Autodesk Fusion 360 part; units mm, degrees
(part 2 of 2)
  spline S44 degree 2 poles (-28.6507, -24.1347) (-29.8115, -24.1371) (-30.4653, -23.6515) knots 0 0 0 1 1 1
  arc A18 (64.0367, -66.674) -> (63.5187, -65.7092) centre (63.7777, -66.1916) ccw
  line L162 (-31.3909, -21.1424) -> (-31.396, -18.6591)
  line L163 (-20.2167, -14.2211) -> (-20.2167, -14.0211)
  line L164 (-32.5375, -24.0363) -> (-33.7962, -24.0388)
  line L165 (-28.678, -21.1369) -> (-31.3909, -21.1424)
  spline S45 degree 5 poles (50.9366, -22.8645) (50.9348, -22.8259) (50.9292, -22.75) (50.9148, -22.6405) (50.8834, -22.5031) (50.8225, -22.3468) (50.738, -22.2071) (50.6282, -22.0855) (50.4922, -21.9825) (50.3313, -21.8972) (50.1475, -21.8281) (49.9836, -21.7847) (49.8519, -21.7585) (49.7602, -21.7438) (49.7134, -21.7371) knots 0 0 0 0 0 0 0.1 0.2 0.3 0.4 0.5 0.6 0.7 0.8 0.9 1 1 1 1 1 1
  line L166 (-18.5375, -12.7629) -> (-18.6809, -12.6194)
  line L167 (48.4274, -26.3644) -> (48.793, -25.0449)
  line L168 (50.9287, -28.6142) -> (49.4213, -28.6142)
  arc A19 (57.5739, -61.8275) -> (56.4337, -61.8275) centre (57.0038, -61.8275) ccw
  line L169 (-17.0167, -15.1211) -> (-17.0167, -14.2211)
  spline S46 degree 2 poles (-33.8519, -19.6208) (-33.9334, -19.2382) (-34.2379, -19.0071) knots 0 0 0 1 1 1
  line L170 (50.0446, -26.3644) -> (48.4274, -26.3644)
  line L171 (-18.9584, -12.7629) -> (-18.8149, -12.6194)
  line L172 (57.0038, -59.0823) -> (51.6038, -59.0823)
  line L173 (51.6038, -60.2085) -> (57.0038, -60.2085)
  spline S47 degree 2 poles (-25.5615, -20.9265) (-25.5595, -21.9003) (-25.9662, -22.658) knots 0 0 0 1 1 1
  line L174 (64.8038, -70.4149) -> (58.1231, -70.4149)
  line L175 (-20.4792, -14.2211) -> (-20.2167, -14.2211)
  line L176 (-17.2792, -14.2211) -> (-17.2792, -14.0211)
  spline S48 degree 2 poles (-29.4415, -18.9209) (-29.8388, -19.0769) (-30.1232, -19.2986) knots 0 0 0 1 1 1
  line L177 (63.7777, -66.1916) -> (60.0038, -68.2176) construction
  line L178 (49.078, -17.2) -> (47.7162, -22.4312)
  spline S49 degree 2 poles (-31.396, -18.6591) (-31.0013, -18.2755) (-30.2513, -17.9827) knots 0 0 0 1 1 1
  spline S50 degree 5 poles (50.9366, -22.8645) (50.9348, -22.8259) (50.9292, -22.75) (50.9148, -22.6405) (50.8834, -22.5031) (50.8225, -22.3468) (50.738, -22.2071) (50.6282, -22.0855) (50.4922, -21.9825) (50.3313, -21.8972) (50.1475, -21.8281) (49.9836, -21.7847) (49.8519, -21.7585) (49.7602, -21.7438) (49.7134, -21.7371) knots 0 0 0 0 0 0 0.1 0.2 0.3 0.4 0.5 0.6 0.7 0.8 0.9 1 1 1 1 1 1
  line L179 (49.4213, -28.6142) -> (50.0446, -26.3644)
  arc A20 (56.4337, -68.8176) -> (57.5739, -68.8176) centre (57.0038, -68.8176) ccw
  line L180 (57.0038, -68.8176) -> (57.0038, -61.8275) construction
  spline S51 degree 2 poles (-28.6528, -23.0589) (-27.8279, -23.0572) (-27.3421, -22.5332) knots 0 0 0 1 1 1
  line L181 (56.4337, -61.8275) -> (56.4337, -68.8176)
  line L182 (-31.3078, -22.3074) -> (-30.0581, -22.071)
  arc A21 (57.0038, -60.2085) -> (57.0038, -59.0823) centre (57.0038, -59.6454) ccw
  line L183 (-17.0167, -15.5211) -> (-17.2792, -15.5211)
  spline S52 degree 2 poles (-25.9662, -22.658) (-26.3729, -23.4158) (-27.1587, -23.8213) knots 0 0 0 1 1 1
  line L184 (50.4816, -66.7499) -> (53.8101, -68.7056)
  arc A22 (58.1231, -70.4149) -> (58.1231, -71.5881) centre (58.1231, -71.0015) ccw
  arc A23 (53.8101, -68.7056) -> (54.5831, -67.39) centre (54.1966, -68.0478) ccw
  spline S53 degree 2 poles (-28.7317, -17.6884) (-27.7537, -17.6864) (-27.0257, -18.0953) knots 0 0 0 1 1 1
  line L185 (52.5226, -22.8607) -> (50.9287, -28.6142)
  spline S54 degree 2 poles (-63.4491, -19.0533) (-63.7208, -19.2728) (-63.7754, -19.5919) knots 0 0 0 1 1 1
  line L186 (-70.944, -17.8799) -> (-65.8795, -17.8697)
  line L187 (-63.8286, -20.6508) -> (-63.8216, -24.0994)
  spline S55 degree 2 poles (-63.7754, -19.5919) (-63.8301, -19.9109) (-63.8286, -20.6508) knots 0 0 0 1 1 1
  line L188 (-65.8795, -17.8697) -> (-65.8773, -19.005)
  line L189 (-69.1434, -23.0556) -> (-66.239, -23.0497)
  line L190 (-66.2369, -24.1043) -> (-70.7996, -24.1135)
  line L191 (-63.8216, -24.0994) -> (-65.0803, -24.1019)
  spline S56 degree 2 poles (-64.6133, -18.4582) (-64.3397, -18.1387) (-63.8808, -17.9485) knots 0 0 0 1 1 1
  line L192 (-66.239, -23.0497) -> (-66.2369, -24.1043)
  line L193 (-65.0803, -24.1019) -> (-65.0869, -20.8277)
  spline S57 degree 2 poles (-65.0869, -20.8277) (-65.0892, -19.7051) (-64.988, -19.2414) knots 0 0 0 1 1 1
  line L194 (-67.3955, -18.923) -> (-70.9419, -18.9302)
  spline S58 degree 2 poles (-64.988, -19.2414) (-64.8869, -18.7776) (-64.6133, -18.4582) knots 0 0 0 1 1 1
  spline S59 degree 2 poles (-62.6416, -18.8327) (-63.1774, -18.8337) (-63.4491, -19.0533) knots 0 0 0 1 1 1
  spline S60 degree 5 poles (-17.0167, -17.9211) (-17.0192, -18.1019) (-17.0247, -18.4483) (-17.0348, -18.9224) (-17.0437, -19.4673) (-17.0058, -20.0268) (-16.8739, -20.4996) (-16.6158, -20.9275) (-16.2341, -21.3563) (-15.7621, -21.8302) (-15.2514, -22.3856) (-14.762, -23.0456) (-14.3504, -23.8136) (-14.0614, -24.6692) (-13.9287, -25.5763) (-13.9743, -26.4898) (-14.2086, -27.362) (-14.6299, -28.1493) (-15.2239, -28.82) (-15.9657, -29.3545) (-16.8219, -29.7417) (-17.7541, -29.9769) (-18.7208, -30.0593) (-19.6804, -29.9888) (-20.5934, -29.7639) (-21.4242, -29.384) (-22.141, -28.8524) (-22.7178, -28.1792) (-23.1347, -27.3841) (-23.3794, -26.5001) (-23.4479, -25.5734) (-23.346, -24.6548) (-23.0896, -23.7924) (-22.7069, -23.0242) (-22.2384, -22.3705) (-21.7396, -21.8252) (-21.2725, -21.3599) (-20.8919, -20.9331) (-20.6344, -20.4981) (-20.5035, -20.0118) (-20.4659, -19.4405) (-20.4724, -18.8956) (-20.4779, -18.4308) (-20.4792, -18.0953) (-20.4792, -17.9211) knots 0 0 0 0 0 0 0.025 0.05 0.075 0.1 0.125 0.15 0.175 0.2 0.225 0.25 0.275 0.3 0.325 0.35 0.375 0.4 0.425 0.45 0.475 0.5 0.525 0.55 0.575 0.6 0.625 0.65 0.675 0.7 0.725 0.75 0.775 0.8 0.825 0.85 0.875 0.9 0.925 0.95 0.975 1 1 1 1 1 1
  line L195 (-16.9853, -15.6382) -> (-17.0481, -20.2041)
  line L196 (-20.4792, -20.1211) -> (-20.4792, -15.7211)
  line L197 (-70.9419, -18.9302) -> (-70.944, -17.8799)
  line L198 (-70.7996, -24.1135) -> (-70.8016, -23.1354)
  line L199 (-51.6345, -24.0748) -> (-54.1432, -17.846)
  spline S61 degree 2 poles (-20.4647, -23.8375) (-20.2015, -23.5818) (-19.7016, -23.3866) knots 0 0 0 1 1 1
  line L200 (-50.9571, -22.6191) -> (-50.1198, -20.3042)
  spline S62 degree 2 poles (-19.5728, -26.1121) (-19.4843, -26.4181) (-19.2415, -26.5948) knots 0 0 0 1 1 1
  circle A24 centre (52.4889, -17.3797) radius 3.1155
  spline S63 degree 2 poles (-17.6398, -27.279) (-18.0391, -27.4868) (-18.6345, -27.488) knots 0 0 0 1 1 1
  spline S64 degree 2 poles (-17.7706, -24.2757) (-18.1002, -23.9064) (-18.6332, -23.9075) knots 0 0 0 1 1 1
  line L201 (-49.735, -19.2531) -> (-49.2233, -17.8361)
  spline S65 degree 2 poles (-17.5512, -23.4617) (-17.0659, -23.7343) (-16.821, -24.2426) knots 0 0 0 1 1 1
  spline S66 degree 2 poles (-16.575, -25.3491) (-16.5737, -25.9983) (-16.8448, -26.5035) knots 0 0 0 1 1 1
  line L202 (-47.8881, -17.8334) -> (-50.3036, -24.0721)
  spline S67 degree 2 poles (-19.7016, -23.3866) (-19.2016, -23.1914) (-18.6885, -23.1904) knots 0 0 0 1 1 1
  line L203 (-60.1094, -24.0919) -> (-61.368, -24.0944)
  line L204 (-54.1432, -17.846) -> (-52.774, -17.8432)
  line L205 (48.765, -61.1704) -> (45.6038, -61.1704) construction
  arc A25 (41.2766, -59.5046) -> (39.9627, -59.5046) centre (40.6197, -59.5046) ccw
  spline S68 degree 2 poles (-17.7621, -26.4203) (-17.4382, -26.0709) (-17.4396, -25.3849) knots 0 0 0 1 1 1
  circle A26 centre (56.0213, -23.5604) radius 3.0414
  line L206 (-60.1161, -20.7666) -> (-60.1094, -24.0919)
  arc A27 (38.4183, -62.0841) -> (36.1328, -68.1777) centre (38.3745, -65.5431) ccw
  line L207 (-65.8773, -19.005) -> (-69.1434, -23.0556)
  line L208 (-59.2311, -18.9066) -> (-59.2332, -17.8562)
  line L209 (-19.6151, -24.7911) -> (-18.6541, -24.7892)
  spline S69 degree 2 poles (-61.3749, -20.7181) (-61.3765, -19.9144) (-61.4237, -19.6764) knots 0 0 0 1 1 1
  line L210 (-50.3036, -24.0721) -> (-51.6345, -24.0748)
  line L211 (40.6197, -66.5435) -> (40.6197, -59.5046) construction
  spline S70 degree 2 poles (-18.6359, -26.7707) (-18.086, -26.7696) (-17.7621, -26.4203) knots 0 0 0 1 1 1
  arc A28 (36.1328, -68.1777) -> (37.0548, -67.0941) centre (36.5938, -67.6359) ccw
  line L212 (-20.4059, -26.2697) -> (-19.5728, -26.1121)
  line L213 (-56.091, -24.0328) -> (-56.1014, -18.9002)
  line L214 (-18.6527, -25.4894) -> (-20.4613, -25.4931)
  line L215 (42.4188, -59.63) -> (44.7886, -66.8332)
  line L216 (-54.8448, -17.8474) -> (-54.8324, -24.0302)
  spline S71 degree 2 poles (-16.821, -24.2426) (-16.5762, -24.751) (-16.575, -25.3491) knots 0 0 0 1 1 1
  line L217 (-49.2233, -17.8361) -> (-47.8881, -17.8334)
  line L218 (-61.368, -24.0944) -> (-61.3749, -20.7181)
  spline S72 degree 5 poles (44.3007, -16.8973) (44.3173, -16.863) (44.3472, -16.7953) (44.3822, -16.6962) (44.409, -16.5691) (44.4071, -16.4191) (44.3671, -16.2787) (44.2861, -16.1486) (44.1636, -16.0291) (44.002, -15.9194) (43.8046, -15.8188) (43.6205, -15.7449) (43.4687, -15.6929) (43.3615, -15.6597) (43.3064, -15.6436) knots 0 0 0 0 0 0 0.1 0.2 0.3 0.4 0.5 0.6 0.7 0.8 0.9 1 1 1 1 1 1
  line L219 (-59.2332, -17.8562) -> (-54.8448, -17.8474)
  line L220 (49.2038, -59.8176) -> (46.3446, -68.6318) construction
  line L221 (-18.6541, -24.7892) -> (-18.6527, -25.4894)
  arc A29 (36.8916, -59.1577) -> (36.0527, -59.6242) centre (36.4722, -59.3909) ccw
  line L222 (46.9604, -68.8315) -> (49.8196, -60.0174)
  circle A30 centre (41.0594, -15.5804) radius 1.0733
  spline S73 degree 2 poles (-19.1617, -24.012) (-19.4265, -24.1161) (-19.6162, -24.2639) knots 0 0 0 1 1 1
  line L223 (35.7794, -15.7004) -> (36.0194, -14.3804)
  line L224 (-19.6162, -24.2639) -> (-19.6151, -24.7911)
  arc A31 (45.7289, -68.432) -> (46.9604, -68.8315) centre (46.3446, -68.6318) ccw
  line L225 (-52.2268, -19.2581) -> (-49.735, -19.2531)
  arc A32 (40.6197, -69.3744) -> (40.6197, -68.2176) centre (40.6197, -68.796) ccw
  spline S74 degree 2 poles (-18.6885, -23.1904) (-18.0365, -23.1891) (-17.5512, -23.4617) knots 0 0 0 1 1 1
  spline S75 degree 2 poles (-18.6345, -27.488) (-19.4084, -27.4895) (-19.8442, -27.1658) knots 0 0 0 1 1 1
  spline S76 degree 2 poles (-61.4237, -19.6764) (-61.5053, -19.2939) (-61.8098, -19.0627) knots 0 0 0 1 1 1
  line L226 (44.5601, -22.3879) -> (42.7329, -22.3879)
  spline S77 degree 2 poles (-19.8442, -27.1658) (-20.28, -26.8421) (-20.4059, -26.2697) knots 0 0 0 1 1 1
  spline S78 degree 2 poles (-35.1102, -17.7013) (-34.2172, -17.6995) (-33.7554, -17.9048) knots 0 0 0 1 1 1
  line L227 (-52.774, -17.8432) -> (-52.2268, -19.2581)
  circle A33 centre (39.0194, -15.5804) radius 0.4327
  line L228 (-54.8324, -24.0302) -> (-56.091, -24.0328)
  line L229 (42.8594, -24.2204) -> (41.6483, -24.5507)
  spline S79 degree 2 poles (-61.8098, -19.0627) (-62.1143, -18.8316) (-62.6416, -18.8327) knots 0 0 0 1 1 1
  line L230 (38.365, -62.7953) -> (36.4722, -59.3909) construction
  spline S80 degree 2 poles (-62.682, -17.7569) (-61.7891, -17.7551) (-61.3273, -17.9604) knots 0 0 0 1 1 1
  arc A34 (44.7886, -66.8332) -> (45.836, -66.4886) centre (45.3123, -66.6609) ccw
  line L231 (-20.4613, -25.4931) -> (-20.4647, -23.8375)
  circle A35 centre (41.0594, -15.5804) radius 0.5367
  arc A36 (38.4003, -63.5068) -> (38.4183, -62.0841) centre (38.4093, -62.7955) ccw
  spline S81 degree 5 poles (35.364, -16.3525) (35.345, -16.369) (35.3063, -16.4012) (35.246, -16.4473) (35.1607, -16.5042) (35.0462, -16.5676) (34.924, -16.6224) (34.7945, -16.6675) (34.6587, -16.7009) (34.5181, -16.7199) (34.3747, -16.7214) (34.231, -16.703) (34.0895, -16.6628) (33.9528, -16.6008) (33.8236, -16.5191) (33.7043, -16.4212) (33.5971, -16.3111) (33.5039, -16.1933) (33.4262, -16.0715) (33.3645, -15.9482) (33.3191, -15.8248) (33.2959, -15.7266) (33.2857, -15.6534) (33.2822, -15.6047) (33.2812, -15.5804) knots 0 0 0 0 0 0 0.05 0.1 0.15 0.2 0.25 0.3 0.35 0.4 0.45 0.5 0.55 0.6 0.65 0.7 0.75 0.8 0.85 0.9 0.95 1 1 1 1 1 1
  spline S82 degree 2 poles (-17.4396, -25.3849) (-17.4411, -24.645) (-17.7706, -24.2757) knots 0 0 0 1 1 1
  arc A37 (38.4003, -63.5068) -> (37.0548, -67.0941) centre (38.3745, -65.5431) ccw
  spline S83 degree 2 poles (-35.8772, -18.9976) (-36.1489, -19.2172) (-36.2036, -19.5362) knots 0 0 0 1 1 1
  spline S84 degree 2 poles (-60.5969, -18.4947) (-60.3284, -18.8237) (-60.2426, -19.185) knots 0 0 0 1 1 1
  line L232 (37.3394, -16.0604) -> (37.8194, -14.5004)
  line L233 (-24.9205, -63.1597) -> (-27.0005, -64.4597) construction
  arc A38 (-24.4038, -63.9865) -> (-25.4373, -62.3329) centre (-24.9205, -63.1597) ccw
  line L234 (-24.1393, -69.2134) -> (-27.7794, -67.1334) construction
  line L235 (-23.6556, -68.3669) -> (-27.2956, -66.2868)
  line L236 (-37.0255, -65.8956) -> (-38.3784, -61.6815)
  arc A39 (-49.9858, -65.6876) -> (-48.5071, -66.1846) centre (-49.2464, -65.9361) ccw
  line L237 (-28.2631, -67.9799) -> (-24.623, -70.0599)
  arc A40 (-24.623, -70.0599) -> (-23.6556, -68.3669) centre (-24.1393, -69.2134) ccw
  line L238 (-41.1451, -59.5878) -> (-45.3305, -59.5878)
  line L239 (-26.4838, -65.2865) -> (-24.4038, -63.9865)
  line L240 (-44.0827, -70.774) -> (-47.9547, -68.0452)
  arc A41 (-46.9952, -61.6857) -> (-48.4739, -61.1888) centre (-47.7345, -61.4372) ccw
  arc A42 (-28.7358, -60.3803) -> (-30.6858, -60.3803) centre (-29.7108, -60.3803) ccw
  line L241 (-29.7108, -64.0124) -> (-29.7108, -60.3803) construction
  arc A43 (-28.6905, -69.3997) -> (-30.5105, -69.3997) centre (-29.6005, -69.3997) ccw
  line L242 (-30.5105, -69.3997) -> (-30.5105, -71.4797)
  line L243 (-42.0828, -71.2842) -> (-38.3358, -68.5989) construction
  line L244 (-28.6905, -71.4797) -> (-28.6905, -69.3997)
  arc A44 (-33.5901, -62.5982) -> (-34.6718, -64.2207) centre (-34.131, -63.4095) ccw
  line L245 (-49.2464, -65.9361) -> (-47.7345, -61.4372) construction
  line L246 (-48.4739, -61.1888) -> (-49.9858, -65.6876)
  line L247 (-25.4373, -62.3329) -> (-27.5173, -63.6329)
  line L248 (-34.6718, -64.2207) -> (-33.1118, -65.2608)
  arc A45 (-41.1451, -61.1478) -> (-41.1451, -59.5878) centre (-41.1451, -60.3678) ccw
  arc A46 (-37.8815, -69.2329) -> (-38.7902, -67.9649) centre (-38.3358, -68.5989) ccw
  line L249 (-32.0301, -63.6383) -> (-33.5901, -62.5982)
  arc A47 (-33.1118, -65.2608) -> (-32.0301, -63.6383) centre (-32.5709, -64.4495) ccw
  arc A48 (-44.9814, -72.0491) -> (-44.0827, -70.774) centre (-44.532, -71.4115) ccw
  line L250 (-34.5019, -70.2048) -> (-30.8619, -67.8647)
  arc A49 (-47.9547, -68.0452) -> (-48.8533, -69.3203) centre (-48.404, -68.6827) ccw
  line L251 (-31.9164, -66.2244) -> (-35.5564, -68.5645)
  line L252 (-48.5071, -66.1846) -> (-46.9952, -61.6857)
  line L253 (-37.7682, -66.134) -> (-39.1211, -61.92) construction
  arc A50 (-35.5564, -68.5645) -> (-34.5019, -70.2048) centre (-35.0291, -69.3846) ccw
  line L254 (-31.3891, -67.0445) -> (-35.0291, -69.3846) construction
  arc A51 (-30.6858, -64.0124) -> (-28.7358, -64.0124) centre (-29.7108, -64.0124) ccw
  arc A52 (-30.8619, -67.8647) -> (-31.9164, -66.2244) centre (-31.3891, -67.0445) ccw
  line L255 (-38.7902, -67.9649) -> (-42.5371, -70.6502)
  line L256 (-29.6005, -71.4797) -> (-29.6005, -69.3997) construction
  line L257 (-48.8533, -69.3203) -> (-44.9814, -72.0491)
  line L258 (-30.6858, -60.3803) -> (-30.6858, -64.0124)
  line L259 (-28.7358, -64.0124) -> (-28.7358, -60.3803)
  line L260 (-45.3305, -61.1478) -> (-41.1451, -61.1478)
  line L261 (-32.5709, -64.4495) -> (-34.131, -63.4095) construction
  arc A53 (-45.3305, -59.5878) -> (-45.3305, -61.1478) centre (-45.3305, -60.3678) ccw
  arc A54 (-38.3784, -61.6815) -> (-39.8637, -62.1584) centre (-39.1211, -61.92) ccw
  arc A55 (-30.5105, -71.4797) -> (-28.6905, -71.4797) centre (-29.6005, -71.4797) ccw
  line L262 (-41.6284, -71.9182) -> (-37.8815, -69.2329)
  arc A56 (-38.5109, -66.3725) -> (-37.0255, -65.8956) centre (-37.7682, -66.134) ccw
  arc A57 (-27.5173, -63.6329) -> (-26.4838, -65.2865) centre (-27.0005, -64.4597) ccw
  line L263 (-39.8637, -62.1584) -> (-38.5109, -66.3725)
  line L264 (-44.532, -71.4115) -> (-48.404, -68.6827) construction
  arc A58 (-42.5371, -70.6502) -> (-41.6284, -71.9182) centre (-42.0828, -71.2842) ccw
  line L265 (-41.1451, -60.3678) -> (-45.3305, -60.3678) construction
  arc A59 (-27.2956, -66.2868) -> (-28.2631, -67.9799) centre (-27.7794, -67.1334) ccw
  line L266 (88.5, -105.5) -> (85.5, -105.5)
  line L267 (85.5, -105.5) -> (85.5, -9.5)
  line L268 (85.5, -9.5) -> (88.5, -9.5)
  line L269 (88.5, -9.5) -> (88.5, -105.5)
  line L270 (-88.5, -9.5) -> (-88.5, -105.5)
  line L271 (-85.5, -105.5) -> (-85.5, -9.5)
  line L272 (28, -111) -> (-28, -111)
  line L273 (-51, -103) -> (-61, -103)
  line L274 (-61, -103) -> (-61, -111)
  line L275 (-61, -111) -> (-51, -111)
  line L276 (-51, -111) -> (-51, -103)
  line L277 (-28, -111) -> (-56, -111)
  line L278 (90, -4) -> (84, -4)
  line L279 (84, -4) -> (84, -4.5)
  line L280 (84, -4.5) -> (90, -4.5)
  line L281 (90, -4.5) -> (90, -4)
  line L282 (90, -111) -> (84, -111)
  line L283 (84, -111) -> (84, -110.5)
  line L284 (84, -110.5) -> (90, -110.5)
  line L285 (90, -110.5) -> (90, -111)
  line L286 (-84, -110.5) -> (-90, -110.5)
  line L287 (-84, -4.5) -> (-90, -4.5)
  line L288 (84, -4.5) -> (-84, -4.5)
  line L289 (-84, -110.5) -> (84, -110.5)
  point P0 (61.02, -25.7233)
  point P1 (46.5762, -56.9164)
  point P2 (46.0215, -56.8133)
  point P3 (46.9394, -27.3404)
  point P4 (33.4994, -16.1804)
  point P5 (-14.3792, -27.6211)
  point P6 (-14.8792, -22.9211)
  point P7 (44.0594, -27.2628)
  point P8 (60.3867, -21.4673)
  point P9 (45.7317, -28.1654)
  point P10 (36.0194, -16.0142)
  point P11 (35.8994, -16.6605)
  point P12 (34.0914, -15.7841)
  point P13 (51.444, -20.7686)
  point P14 (63.9087, -20.9288)
  point P15 (44.7794, -28.5404)
  point P16 (37.3394, -16.6604)
  point P17 (43.4594, -28.3004)
  point P18 (34.8065, -16.6605)
  point P19 (57.9901, -18.9866)
  point P20 (-20.7292, -20.6211)
  point P21 (-22.5675, -22.8627)
  point P22 (-18.7792, -30.0211)
  point P23 (-22.9792, -27.6211)
  point P24 (-16.7792, -20.6211)
  point P25 (34.3141, -16.0142)
  point P26 (36.4355, -16.0142)
  point P27 (52.3172, -21.7688)
  point P28 (34.8282, -15.7841)
  point P29 (37.413, -16.3545)
  point P30 (50.6346, -22.1023)
  point P31 (44.9249, -27.2628)
  point P32 (34.0994, -16.6605)
  point P33 (44.3007, -16.184)
  point P34 (45.922, -16.1545)
  point P35 (48.6673, -15.0707)
  point P36 (47.4568, -16.2272)
  point P37 (58.4309, -20.5116)
  point P38 (50.6346, -22.1023)
  point P39 (60.5566, -20.5116)
  point P40 (56.7906, -20.1404)
  point P41 (49.078, -16.1977)
  point P42 (49.8965, -23.22)
  point P43 (45.5113, -15.0275)
  point P44 (46.5762, -56.9164)
  point P45 (49.267, -68.4427)
  point P46 (46.5762, -56.9164)
  point P47 (62.2394, -20.5807)
  point P48 (36.4573, -16.6605)
  point P49 (59.5394, -24.3404)
  point P50 (-33.2091, -68.2146)
  point P51 (-48.4905, -63.6867)
  point P52 (-29.7108, -62.1964)
  point P53 (-46.468, -70.0471)
  point P54 (-38.4446, -64.027)
  point P55 (-33.3509, -63.9295)
  point P56 (-40.2093, -69.9415)
  point P57 (-25.9605, -63.8097)
  point P58 (-29.6005, -70.4397)
  point P59 (-36.6222, -66.278)
  point P60 (-25.9593, -68.1734)
  point P61 (-43.2378, -60.3678)
  dimension "d154" = 180
  dimension "d155" = 115
  dimension "d156" = 180
  dimension "d157" = 4
  dimension "d158" = 1.5
  dimension "d159" = 5.5
  dimension "d160" = 3
  dimension "d161" = 1.5
  dimension "d162" = 1.5
  dimension "d163" = 5.5
  dimension "d164" = 3
  dimension "d165" = 56
  dimension "d166" = 10
  dimension "d167" = 8
  dimension "d168" = 0.5
  dimension "d169" = 0.5
  constraint horizontal L4
  constraint vertical L5
  constraint horizontal L6
  constraint vertical L7
  constraint coincident L0.end L1.start
  constraint horizontal L8
  constraint vertical L9
  constraint horizontal L10
  constraint vertical L11
  constraint perpendicular L5 L12
  constraint perpendicular L10 L13
  constraint perpendicular L13 L14
  constraint coincident L10 L15.end
  constraint perpendicular L10 L15
  constraint coincident L10 L16.end
  constraint coincident L2 L17.end
  constraint perpendicular L2 L17
  constraint coincident L2.end L3.start
  constraint coincident L2 L18.end
  constraint perpendicular L18 L19
  constraint perpendicular L19 L20
  constraint coincident L2 L21.end
  constraint perpendicular L2 L21
  constraint symmetric L12.end L23 L28.start
  constraint symmetric L13.end L23 L27.start
  constraint symmetric L14.end L23 L26.start
  constraint symmetric L15.end L23 L25.start
  constraint symmetric L16.end L23 L24.start
  constraint symmetric L17.end L23 L24.end
  constraint symmetric L2.end L23 L1.end
  constraint symmetric L18.end L23 L29.end
  constraint symmetric L19.end L23 L30.end
  constraint symmetric L20.end L23 L31.end
  constraint symmetric L21.end L23 L32.end
  constraint parallel L179 L185
  constraint parallel L168 L170
  constraint parallel L167 L185
  constraint parallel L156 L170
  constraint parallel L142 L167
  constraint perpendicular L117 L123
  constraint perpendicular L93 L117
  constraint perpendicular L88 L229
  constraint perpendicular L56 L229
  constraint concentric A30 A35
  constraint coincident L79.start A35
  constraint coincident L79.end A30
  constraint coincident L106.start A35
  constraint coincident L106.end A30
  constraint perpendicular L79 L106
  constraint concentric A0 A33
  constraint parallel L71 L232
  constraint parallel L101 L223
  constraint parallel L57 L59
  constraint parallel L58 L101
  constraint midpoint P49 L68
  constraint tangent L145 A17
  constraint tangent L127 A17
  constraint parallel L127 L145
  constraint tangent L127 A15
  constraint tangent A15 L145
  constraint tangent A4 L83
  constraint tangent A4 L76
  constraint parallel L76 L83
  constraint tangent L76 A11
  constraint tangent L83 A11
  constraint tangent L121 A16
  constraint tangent A16 L184
  constraint parallel L121 L184
  constraint tangent L184 A23
  constraint tangent L121 A23
  constraint tangent L134 A19
  constraint tangent A19 L181
  constraint parallel L134 L181
  constraint tangent A20 L181
  constraint tangent L134 A20
  constraint tangent A14 L150
  constraint tangent A14 L147
  constraint parallel L147 L150
  constraint tangent L147 A18
  constraint tangent L150 A18
  constraint tangent L89 A12
  constraint tangent A12 L174
  constraint parallel L89 L174
  constraint tangent L174 A22
  constraint tangent L89 A22
  constraint perpendicular L126 L134
  constraint tangent A13 L172
  constraint tangent A13 L173
  constraint parallel L172 L173
  constraint tangent L173 A21
  constraint tangent L172 A21
  constraint perpendicular L130 L134
  constraint tangent L116 A31
  constraint tangent L222 A31
  constraint parallel L116 L222
  constraint tangent A9 L222
  constraint tangent A9 L116
  constraint tangent L80 A10
  constraint tangent L55 A10
  constraint parallel L55 L80
  constraint tangent L55 A5
  constraint tangent A5 L80
  constraint coincident A5.centre L220
  constraint tangent A1 L105
  constraint tangent A1 L215
  constraint parallel L105 L215
  constraint tangent L215 A34
  constraint tangent L105 A34
  constraint tangent L110 A25
  constraint tangent L61 A25
  constraint parallel L61 L110
  constraint tangent L61 A6
  constraint tangent A6 L110
  constraint tangent A3 L48
  constraint tangent L35 A3
  constraint parallel L35 L48
  constraint tangent L35 A32
  constraint tangent L48 A32
  constraint tangent A27 A36
  constraint tangent A36 A37
  constraint tangent A28 A37
  constraint tangent A27 A28
  constraint tangent L78 A29
  constraint tangent L64 A29
  constraint parallel L64 L78
  constraint tangent A2 L64
  constraint tangent A2 L78
  constraint coincident A2.centre A7
  constraint midpoint L109.end L196
  constraint midpoint L109.start L195
  constraint perpendicular L109 L196
  constraint coincident L45.end L196
  constraint perpendicular L45 L196
  constraint coincident L91.end L196
  constraint perpendicular L45 L113
  constraint perpendicular L115 L196
  constraint perpendicular L84 L115
  constraint perpendicular L84 L100
  constraint perpendicular L95 L100
  constraint perpendicular L95 L183
  constraint perpendicular L100 L124
  constraint perpendicular L124 L131
  constraint perpendicular L131 L169
  constraint perpendicular L124 L161
  constraint perpendicular L161 L176
  constraint parallel L146 L152
  constraint parallel L155 L159
  constraint parallel L125 L144
  constraint parallel L141 L157
  constraint parallel L159 L171
  constraint perpendicular L166 L171
  constraint parallel L151 L152
  constraint parallel L86 L148
  constraint parallel L43 L77
  constraint tangent A42 L259
  constraint tangent A42 L258
  constraint parallel L258 L259
  constraint tangent A51 L258
  constraint tangent A51 L259
  constraint midpoint P52 L241
  constraint tangent A44 L249
  constraint tangent A44 L248
  constraint parallel L248 L249
  constraint tangent L248 A47
  constraint tangent L249 A47
  constraint midpoint P55 L261
  constraint tangent L251 A50
  constraint tangent L250 A50
  constraint parallel L250 L251
  constraint tangent L250 A52
  constraint tangent L251 A52
  constraint midpoint P50 L254
  constraint tangent A43 L244
  constraint tangent A43 L242
  constraint parallel L242 L244
  constraint tangent L242 A55
  constraint tangent L244 A55
  constraint midpoint P58 L256
  constraint tangent L235 A59
  constraint tangent L237 A59
  constraint parallel L235 L237
  constraint tangent L237 A40
  constraint tangent L235 A40
  constraint midpoint P60 L234
  constraint tangent L247 A57
  constraint tangent L239 A57
  constraint parallel L239 L247
  constraint tangent A38 L239
  constraint tangent A38 L247
  constraint midpoint P57 L233
  constraint tangent A46 L262
  constraint tangent A46 L255
  constraint parallel L255 L262
  constraint tangent L255 A58
  constraint tangent L262 A58
  constraint midpoint P56 L243
  constraint tangent L236 A54
  constraint tangent A54 L263
  constraint parallel L236 L263
  constraint tangent A56 L263
  constraint tangent L236 A56
  constraint midpoint P54 L253
  constraint tangent L238 A53
  constraint tangent L260 A53
  constraint parallel L238 L260
  constraint tangent A45 L260
  constraint tangent L238 A45
  constraint midpoint P61 L265
  constraint tangent A41 L252
  constraint tangent A41 L246
  constraint parallel L246 L252
  constraint tangent A39 L246
  constraint tangent A39 L252
  constraint midpoint P51 L245
  constraint tangent L240 A49
  constraint tangent A49 L257
  constraint parallel L240 L257
  constraint tangent A48 L257
  constraint tangent L240 A48
  constraint midpoint P53 L264
  constraint horizontal L266
  constraint vertical L267
  constraint horizontal L268
  constraint vertical L269
  constraint symmetric L23 L14.end L26.start
  constraint symmetric L23 L19.end L30.end
  constraint horizontal L272
  constraint midpoint L10 L272
  constraint horizontal L273
  constraint vertical L274
  constraint horizontal L275
  constraint vertical L276
  constraint midpoint L275 L277.end
  constraint parallel L275 L277
  constraint horizontal L278
  constraint vertical L279
  constraint horizontal L280
  constraint vertical L281
  constraint horizontal L282
  constraint vertical L283
  constraint horizontal L284
  constraint vertical L285
  constraint symmetric L23 L279.end L287.start
  constraint symmetric L23 L280.end L287.end
  constraint symmetric L23 L283.end L286.start
  constraint symmetric L23 L284.end L286.end
  measures "d154" distance of L0.end L0.start
  measures "d155" distance of L0.end L6.end
  measures "d156" distance of L6.end L5.end
  measures "d157" distance of L6.end L10.end
  measures "d158" distance of L9.end L12.end
  measures "d159" distance of L12.end L13.end
  measures "d160" distance of L13.end L14.end
  measures "d161" distance of L15.end L16.end
  measures "d162" distance of L2.end L18.end
  measures "d163" distance of L18.end L19.end
  measures "d164" distance of L19.end L20.end
  measures "d165" distance of L272.start L272.end
  measures "d166" distance of L273.start L273.end
  measures "d167" distance of L273.start L275.end
  measures "d168" distance of L2.end L280.end
  measures "d169" distance of L9.end L284.end
extrude "Extrusão1'" add sketch "Esboço11" against normal blind 57.5 separate body contours L5 L13 L19 L269 L280 L284 | L7 L28 L30 L270 L286 L287 | L15 L17 L21 L267 L280 L284 | L24 L26 L32 L271 L286 L287 makes body 4 at (-85.5, 75.1667, 60.8333) makes body 5 at (84, 75.1667, 60.8333) makes body 6 at (-90, 39.8333, 60.8333) makes body 7 at (88.5, 39.8333, 60.8333) in component "Component"
extrude "Extrusão2'" add sketch "Esboço11" against normal blind 52 contours L14 L20 L266 L267 L268 L269 | L27 L31 L270 L271 bodies 4 5 6 7 in component "Component"
extrude "Extrusão3'" add sketch "Esboço11" against normal blind 4 contours L5 L13 L19 L269 L280 L284 | L7 L28 L30 L270 L286 L287 | L19 L20 L21 L268 L280 | L30 L31 L32 L287 | L15 L17 L21 L267 L280 L284 | L14 L20 L266 L267 L268 L269 | L13 L14 L15 L266 L284 | L24 L26 L32 L271 L286 L287 | L27 L31 L270 L271 | L26 L27 L28 L286 | L17 L24 L273 L274 L276 L288 L289 | S0 S10 S13 S54 L187 S55 L191 S56 L193 S57 S58 S59 L203 L206 S69 L218 S76 S79 S80 S84 | L34 L186 L188 L189 L190 L192 L194 L197 L198 L207 | L35 A3 L48 A32 | A0 A30 | A0 L79 L106 A30 A35 | A0 A30 | L79 L106 A30 A35 | A35 | L36 L44 L54 L65 L74 L92 L96 L97 L98 L99 L102 L108 L118 | S1 S4 S5 L49 L66 L82 S15 S16 S22 L120 S24 S27 S33 L132 S40 S41 L164 S46 S78 S83 | S2 L39 S6 L57 L58 L59 L71 S14 L85 L101 S20 S21 L223 S81 L232 | L37 L53 S12 L70 | A1 L105 L215 A34 | L38 L63 L200 | S3 L42 L52 S7 L107 L111 L112 S19 | L40 L50 L87 L91 L196 | L40 L45 L47 L50 L81 L84 L87 L91 L95 L100 L113 L115 L124 L125 L131 L135 L136 L137 L139 L146 L155 L161 L163 L169 L175 L176 L183 L196 | L41 L46 L62 L104 S25 S72 L226 | L43 L75 L77 L94 L114 | A2 L64 L78 A27 A36 | A2 L64 L78 A27 A28 A36 A37 | L64 L78 A27 A29 A36 | A4 L76 L83 A11 | L55 L80 A10 L116 | L55 A5 L80 L116 L222 | L55 A5 L116 L222 A31 | A5 L80 A9 L116 L222 | A5 L222 | L56 L88 L93 S18 L117 L123 S26 S31 L143 L229 | S8 S9 S11 S61 S62 S63 S64 S65 S66 S67 S68 L209 S70 L212 L214 S71 L221 S73 L224 S74 S75 S77 L231 S82 | L60 L69 L72 L103 | L61 A6 L110 A25 | L67 L208 L213 L216 L219 L228 | A8 | L86 L90 L148 L149 | S17 S28 S29 S30 S32 S34 S35 L133 L138 S37 S38 L154 S39 S43 S44 L162 L165 S47 S48 S49 S51 L182 S52 S53 | L89 A12 L174 A22 | L109 S60 L195 | S60 L196 | S23 L129 L140 S42 L158 L160 L178 | L121 A16 L184 A23 | L122 S36 L142 L156 S45 L167 L168 L170 S50 L179 L185 | A13 L172 L173 A21 | A14 L147 L150 A18 | L127 A15 L145 A17 | L134 A19 A20 L181 | L141 L151 L166 L171 | L144 L152 L157 L159 | L199 L201 L202 L204 L210 L217 L225 L227 | A24 | A26 | A33 | A38 L239 L247 A57 | L235 L237 A40 A59 | L236 A54 A56 L263 | A39 A41 L246 L252 | L238 A45 L260 A53 | L240 A48 A49 L257 | A42 A51 L258 L259 | A43 L242 L244 A55 | A44 L248 L249 A47 | A46 L255 L262 A58 | L250 L251 A50 A52 bodies 4 5 in component "Component"
extrude "Extrusão4'" cut sketch "Esboço11" against normal blind 1 contours S0 S10 S13 S54 L187 S55 L191 S56 L193 S57 S58 S59 L203 L206 S69 L218 S76 S79 S80 S84 | L34 L186 L188 L189 L190 L192 L194 L197 L198 L207 | L35 A3 L48 A32 | A0 A30 | A0 L79 L106 A30 A35 | A0 A30 | L79 L106 A30 A35 | A35 | L36 L44 L54 L65 L74 L92 L96 L97 L98 L99 L102 L108 L118 | S1 S4 S5 L49 L66 L82 S15 S16 S22 L120 S24 S27 S33 L132 S40 S41 L164 S46 S78 S83 | S2 L39 S6 L57 L58 L59 L71 S14 L85 L101 S20 S21 L223 S81 L232 | L37 L53 S12 L70 | A1 L105 L215 A34 | L38 L63 L200 | S3 L42 L52 S7 L107 L111 L112 S19 | L40 L45 L47 L50 L81 L84 L87 L91 L95 L100 L113 L115 L124 L125 L131 L135 L136 L137 L139 L146 L155 L161 L163 L169 L175 L176 L183 L196 | L41 L46 L62 L104 S25 S72 L226 | L43 L75 L77 L94 L114 | A2 L64 L78 A27 A36 | A2 L64 L78 A27 A28 A36 A37 | L64 L78 A27 A29 A36 | A4 L76 L83 A11 | L55 L80 A10 L116 | L55 A5 L80 L116 L222 | L55 A5 L116 L222 A31 | A5 L80 A9 L116 L222 | A5 L222 | L56 L88 L93 S18 L117 L123 S26 S31 L143 L229 | S8 S9 S11 S61 S62 S63 S64 S65 S66 S67 S68 L209 S70 L212 L214 S71 L221 S73 L224 S74 S75 S77 L231 S82 | L60 L69 L72 L103 | L61 A6 L110 A25 | L67 L208 L213 L216 L219 L228 | A8 | L86 L90 L148 L149 | S17 S28 S29 S30 S32 S34 S35 L133 L138 S37 S38 L154 S39 S43 S44 L162 L165 S47 S48 S49 S51 L182 S52 S53 | L89 A12 L174 A22 | L109 S60 L195 | S23 L129 L140 S42 L158 L160 L178 | L121 A16 L184 A23 | L122 S36 L142 L156 S45 L167 L168 L170 S50 L179 L185 | A13 L172 L173 A21 | A14 L147 L150 A18 | L127 A15 L145 A17 | L134 A19 A20 L181 | L141 L151 L166 L171 | L144 L152 L157 L159 | L199 L201 L202 L204 L210 L217 L225 L227 | A24 | A26 | A33 | A38 L239 L247 A57 | L235 L237 A40 A59 | L236 A54 A56 L263 | A39 A41 L246 L252 | L238 A45 L260 A53 | L240 A48 A49 L257 | A42 A51 L258 L259 | A43 L242 L244 A55 | A44 L248 L249 A47 | A46 L255 L262 A58 | L250 L251 A50 A52 bodies 4 in component "Component"
component "Component" placed x (1, 0, 0) y (0, 1, 0) z (0, 0, 1) at (0, 0, 0)
equation "d115 = -4.00 mm - 5 mm"
equation "d172 = -48 mm - 4 mm"
